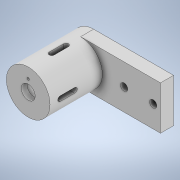
# Autodesk Inventor part: bearing_mount3
Saved by Autodesk Inventor 2022.3 (Build 263350000, 350)
## iProperties
Created: 2022-01-28
Part Number: bearing_mount3
Material: Generic
Document SubType Name: Modeling
Designer: Martijn
Density: 1 g/cm^3
Appearance: Default
Author: Martijn
Autodesk Inventor part; units mm, degrees
ref_plane "YZ Plane" through (0, 0, 0) normal (1, 0, 0) x (0, 1, 0)
ref_plane "XZ Plane" through (0, 0, 0) normal (0, 1, 0) x (-1, 0, 0)
ref_plane "XY Plane" through (0, 0, 0) normal (0, 0, 1) x (1, 0, 0)
sketch "Sketch1" plane through (0, 0, 0) normal (0, 0, 1) x (1, 0, 0)
  line L0 (15, 15) -> (70, 15)
  line L1 (70, 15) -> (70, -15)
  line L2 (70, -15) -> (15, -15)
  line L3 (-14, 0) -> (84, 0) projected
  arc A0 (15, 15) -> (15, -15) centre (15, 0) ccw
  line L4 (0, -21) -> (0, 21) projected
  line L5 (15, 0) -> (70, 0)
  point P0 (0, 0)
  dimension "d4" = 30
  dimension "d15" = 15
  dimension "d16" = 55
  constraints: 8 end point, 2 parallel, 2 point on circle, 1 centre point, 1 midpoint, 1 perpendicular, 1 point on line, 1 tangent, 1 vertical
  measures "d4" distance between parallel lines of L2 L0
  measures "d15" radius of A0
  measures "d16" distance from line of L1 L5.start
extrude "Extrusion1" add sketch "Sketch1" along normal blind 9
sketch "Sketch2" plane through (0, 0, 9) normal (0, 0, 1) x (1, 0, 0)
  circle A0 centre (15, 0) radius 11
  arc A1 (15, 15) -> (15, -15) centre (15, 0) ccw projected
  point P0 (0, 0)
  dimension "d7" = 22
  constraints: 1 centre point, 1 concentric
  measures "d7" diameter of A0
extrude "Extrusion2" cut sketch "Sketch2" against normal blind 10
sketch "Sketch3" plane through (0, 0, 9) normal (0, 0, 1) x (1, 0, 0)
  circle A0 centre (45, 0) radius 2.5
  circle A1 centre (65, 0) radius 2.5
  line L0 (70, -15) -> (70, 15) projected
  point P0 (0, 0)
  dimension "d28" = 3.4
  dimension "d29" = 7
  dimension "d30" = 10
  dimension "d31" = 15
  dimension "d10" = 5
  dimension "d11" = 5
  dimension "d12" = 25
  constraints: 2 centre point, 1 equal radius
  measures "d10" diameter of A0
  measures "d11" distance from line of L0 A1.centre
  measures "d12" distance from line of L0 A0.centre
extrude "Extrusion3" cut sketch "Sketch3" against normal blind 25
sketch "Sketch4" plane through (0, 0, 9) normal (0, 0, 1) x (1, 0, 0)
  circle A0 centre (15, 0) radius 15
  circle A1 centre (15, 0) radius 11
  circle A2 centre (15, 0) radius 11 projected
  arc A3 (15, 15) -> (15, -15) centre (15, 0) ccw projected
  point P0 (0, 0)
  constraints: 4 concentric, 2 centre point
extrude "Extrusion4" add sketch "Sketch4" along normal blind 0.001
sketch "Sketch5" plane through (15, 0, 9.001) normal (0, 0, 1) x (1, 0, 0)
  circle A0 centre (0, 0) radius 15
  circle A1 centre (0, 0) radius 10.5
  circle A2 centre (0, 0) radius 15 projected
  point P0 (-15, 0)
  dimension "d19" = 21
  constraints: 2 centre point, 1 coincident, 1 horizontal alignment, 1 other
  measures "d19" diameter of A1
extrude "Extrusion5" add sketch "Sketch5" along normal blind 32
sketch "Sketch6" plane through (15, 0, 41.001) normal (0, 0, 1) x (1, 0, 0)
  circle A0 centre (0, 0) radius 4.8
  circle A1 centre (0, 0) radius 15
  circle A2 centre (0, 0) radius 15 projected
  point P0 (-15, 0)
  dimension "d22" = 9.6
  constraints: 2 centre point, 1 coincident, 1 horizontal alignment, 1 other
  measures "d22" diameter of A0
extrude "Extrusion6" add sketch "Sketch6" along normal blind 4
sketch "Sketch7" plane through (70, -15, 0) normal (1, 0, 0) x (0, 0, -1)
  line L0 (-45.001, 30) -> (-45.001, 0) projected
  arc A0 (-38.001, 16.7) -> (-38.001, 13.3) centre (-38.001, 15) ccw
  line L1 (-38.001, 16.7) -> (-28.001, 16.7)
  arc A1 (-28.001, 13.3) -> (-28.001, 16.7) centre (-28.001, 15) ccw
  line L2 (-38.001, 13.3) -> (-28.001, 13.3)
  line L3 (-9, 0) -> (-9, 30) projected
  line L4 (0, 0) -> (-9, 0) projected
  point P0 (0, 15)
  dimension "d28" = 3.4
  dimension "d29" = 7
  dimension "d30" = 10
  dimension "d31" = 15
  constraints: 4 end point, 4 point on circle, 4 tangent, 2 centre point, 1 parallel, 1 perpendicular
  measures "d28" distance between parallel lines of L2 L1
  measures "d29" distance from line of L0 A0.centre
  measures "d30" distance of A0.centre A1.centre
  measures "d31" distance from line of L4 A1.centre
extrude "Extrusion7" cut sketch "Sketch7" against normal blind 50
sketch "Sketch8" plane through (15, 15, 0) normal (0, 1, 0) x (1, 0, 0)
  arc A0 (-1.7, -29.001) -> (1.7, -29.001) centre (0, -29.001) ccw
  arc A1 (1.7, -19.001) -> (-1.7, -19.001) centre (0, -19.001) ccw
  line L0 (-1.7, -29.001) -> (-1.7, -19.001)
  line L1 (1.7, -19.001) -> (1.7, -29.001)
  line L2 (0, -29.001) -> (0, -19.001)
  line L3 (55, -9) -> (0, -9) projected
  line L4 (55, 0) -> (55, -9) projected
  line L5 (-15, -45.001) -> (15, -45.001) projected
  point P0 (-15, 0)
  dimension "d34" = 55
  dimension "d35" = 3.4
  dimension "d36" = 16
  dimension "d37" = 10
  constraints: 6 end point, 4 point on circle, 4 tangent, 2 centre point, 1 parallel, 1 perpendicular
  measures "d34" distance between parallel lines of L4 L2
  measures "d35" distance between parallel lines of L1 L0
  measures "d36" distance from line of L5 L2.start
  measures "d37" distance of L2.end L2.start
extrude "Extrusion8" cut sketch "Sketch8" against normal blind 20
sketch "Sketch9" plane through (15, -15, 0) normal (0, -1, 0) x (1, 0, 0)
  arc A0 (-1.7, 11.001) -> (1.7, 11.001) centre (0, 11.001) ccw
  line L0 (-1.7, 11.001) -> (-1.7, 21.001)
  line L1 (1.7, 11.001) -> (1.7, 21.001)
  arc A1 (1.7, 21.001) -> (-1.7, 21.001) centre (0, 21.001) ccw
  line L2 (15, 45.001) -> (-15, 45.001) projected
  line L3 (55, 0) -> (55, 9) projected
  point P0 (-15, 0)
  dimension "d40" = 24
  dimension "d41" = 10
  dimension "d42" = 3.4
  dimension "d43" = 55
  constraints: 4 end point, 4 point on circle, 4 tangent, 2 centre point, 2 vertical
  measures "d40" distance from line of L2 A1.centre
  measures "d41" distance of A1.centre A0.centre
  measures "d42" distance between parallel lines of L1 L0
  measures "d43" distance from line of L3 A0.centre
extrude "Extrusion9" cut sketch "Sketch9" against normal blind 20
sketch "Sketch10" plane through (15, 0, 45.001) normal (0, 0, 1) x (1, 0, 0)
  circle A0 centre (0, 7.92) radius 0.85
  circle A1 centre (0, 0) radius 15 projected
  line L0 (0, 7.92) -> (0, 0)
  point P0 (-15, 0)
  dimension "d46" = 1.7
  dimension "d47" = 7.92
  constraints: 2 end point, 1 centre point, 1 coincident, 1 horizontal alignment, 1 vertical
  measures "d46" diameter of A0
  measures "d47" distance of point (0, 0) L0.start
extrude "Extrusion10" cut sketch "Sketch10" against normal blind 1.8 contours A0
equation "\"d13\" = d12"
body "Solid1"
